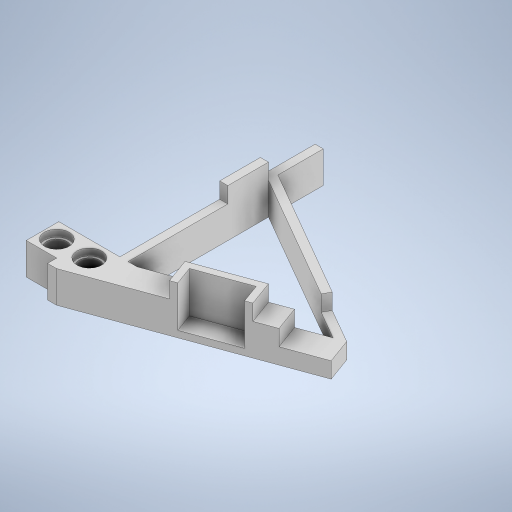
# Autodesk Inventor part: blokerv9
Saved by Autodesk Inventor 2023 (Build 270158000, 158)
## iProperties
Created: 2022-10-20
Part Number: blokerv9
Material: Ogólny
Document SubType Name: Modeling
Designer: kamil
Density: 1 g/cm^3
Appearance: Domyślna
Author: kamil
Autodesk Inventor part; units mm, degrees
ref_plane "YZ Plane" through (0, 0, 0) normal (1, 0, 0) x (0, 1, 0)
ref_plane "XZ Plane" through (0, 0, 0) normal (0, 1, 0) x (-1, 0, 0)
ref_plane "XY Plane" through (0, 0, 0) normal (0, 0, 1) x (1, 0, 0)
sketch "Sketch2" plane through (0, 0, 0) normal (0, 1, 0) x (-1, 0, 0)
  line L0 (7.5, -4) -> (-7.5, -4)
  line L1 (-7.5, -4) -> (-7.5, 4)
  line L2 (-7.5, 4) -> (7.5, 4)
  line L3 (7.5, 4) -> (7.5, -4)
  circle A0 centre (4, 0) radius 2.5
  circle A1 centre (-4, 0) radius 2.5
  line L4 (0, -4) -> (0, 11) construction
  circle A2 centre (0, 11) radius 3.7 construction
  line L5 (-30.3941, -4) -> (1.2655, 7.5231) construction
  line L6 (-17.5, -4) -> (-17.5, 0.6931)
  line L7 (-17.5, 0.6931) -> (0, 7.0625)
  line L8 (0, 7.0625) -> (0, 4)
  line L9 (-17.5, -4) -> (-7.5, -4)
  line L10 (-11.8902, 2.7349) -> (-12.4882, 4.3778) construction
  line L11 (-17.5, 0.6931) -> (-51.6831, -11.7486)
  line L12 (-51.6831, -11.7486) -> (-49.4993, -17.7486)
  circle A3 centre (0, 7.0625) radius 55 construction
  line L13 (0, 14.7) -> (0, 62.0625) construction
  line L14 (-49.4993, -17.7486) -> (-11.7254, -4)
  line L15 (-7.5, -4) -> (-7.5, -41.9969)
  line L16 (-7.5, -41.9969) -> (-49.4993, -17.7486)
  line L17 (-9.5, -4) -> (-9.5, -38.5328)
  line L18 (-9.5, -38.5328) -> (-47.0459, -16.8556)
  line L19 (0, 6.2625) -> (-2.198, 6.2625)
  line L20 (-22.5526, -1.1459) -> (-20.3688, -7.1459)
  line L21 (-20.3688, -7.1459) -> (-35.4039, -12.6183)
  line L22 (-35.4039, -12.6183) -> (-37.5877, -6.6183)
  line L23 (-37.5877, -6.6183) -> (-22.5526, -1.1459)
  line L24 (-9.5, -38.5328) -> (-9.5, -51.9969)
  line L25 (-9.5, -51.9969) -> (-7.5, -51.9969)
  line L26 (-7.5, -51.9969) -> (-7.5, -41.9969)
  arc A4 (0, 47.0625) -> (-37.5877, -6.6183) centre (0, 7.0625) ccw construction
  line L27 (-7.5, -38.5328) -> (-9.5, -38.5328)
  line L28 (-9.5, -38.5328) -> (-9.5, -28.5328)
  line L29 (-9.5, -28.5328) -> (-7.5, -28.5328)
  line L30 (-7.5, -28.5328) -> (-7.5, -38.5328)
  circle A5 centre (4, 0) radius 3.05
  circle A6 centre (-4, 0) radius 3.05
  line L31 (-42.2862, -8.3284) -> (-40.1023, -14.3284)
  line L32 (-40.1023, -20.8645) -> (-41.1023, -22.5965)
  point P0 (0, 0)
  point P1 (7.5, 0)
  point P2 (0, 3.5)
  point P3 (-9.5, -40.8422)
  dimension "d6" = 5
  dimension "d7" = 8
  dimension "d9" = 11
  dimension "d10" = 7.4
  dimension "d11" = 8
  dimension "d12" = 15
  dimension "d13" = 70
  dimension "d14" = 10
  dimension "d21" = 14
  dimension "d25" = 55
  dimension "d27" = 6
  dimension "d35" = 60
  dimension "d36" = 3.5
  dimension "d37" = 2
  dimension "d38" = 2
  dimension "d39" = 0.8
  dimension "d40" = 10
  dimension "d41" = 40
  dimension "d42" = 16
  dimension "d43" = 10
  dimension "d46" = 6.1
  dimension "d47" = 6.1
  dimension "d50" = 10
  constraints: 66 end point, 20 point on line, 12 perpendicular, 8 parallel, 7 centre point, 6 point on circle, 5 coincident, 5 vertical, 4 midpoint, 3 horizontal alignment, 3 vertical alignment, 2 horizontal, 1 collinear, 1 tangent, 1 other
  measures "d6" diameter of A0
  measures "d7" distance of A1.centre A0.centre
  measures "d9" distance of L4.end point (0, 0)
  measures "d10" diameter of A2
  measures "d11" distance of L2.end L0.start
  measures "d12" distance of L0.start L0.end
  measures "d13" angle of L4 L5
  measures "d14" distance of L6.start L0.end
  measures "d21" distance of L10.start L5.end
  measures "d25" distance of L13.end L7.end
  measures "d27" vertical distance of L11.end L12.end
  measures "d35" angle of L16 L15
  measures "d36" horizontal distance of L15.start A1.centre
  measures "d37" distance between parallel lines of L16 L18
  measures "d38" distance between parallel lines of L17 L15
  measures "d39" distance of L7.end L19.start
  measures "d40" distance of L25.end L15.end
  measures "d41" distance of A4.start A4.centre
  measures "d42" distance between parallel lines of L20 L22
  measures "d43" distance of L29.end L27.start
  measures "d46" diameter of A5
  measures "d47" diameter of A6
  measures "d50" distance from line of L11.end L31
extrude "Extrusion1" add sketch "Sketch2" along normal blind 7.8 contours L0 L1 L2 L3 | L9 L6 L7 L19 L8 L2 L1 | L15 L29 L17 L9 | L14 L20 L11 L6 L9 | L15 L16 L24 L27 | L24 L16 L32 L18 | L26 L25 L24 L16 | L14 L31 L11 L22
extrude "Wyciągnięcie proste3" add sketch "Sketch2" along normal blind 11.7 contours L15 L27 L17 L29 | L14 L22 L11 L20
extrude "Wyciągnięcie proste4" add sketch "Sketch2" along normal blind 6.1 contours A5 | A6
extrude "Wyciągnięcie proste5" add sketch "Sketch2" along normal blind 3.9 contours L32 L16 L14 L18 | L14 L12 L11 L31
sketch "Szkic6" plane through (2.198, 0, 6.2625) normal (0.342, 0, 0.9397) x (0.9397, 0, -0.342)
  line L0 (21.661, 11.7) -> (37.661, 11.7) projected
  line L1 (23.261, 11.7) -> (36.061, 11.7)
  line L2 (36.061, 11.7) -> (36.061, 1.6)
  line L3 (36.061, 1.6) -> (23.261, 1.6)
  line L4 (23.261, 1.6) -> (23.261, 11.7)
  line L5 (37.661, 7.8) -> (37.661, 11.7) projected
  line L6 (21.661, 7.8) -> (21.661, 11.7) projected
  line L7 (0, 0) -> (52.661, 0) projected
  point P0 (0.0765, 0)
  point P1 (37.661, 9.75)
  point P2 (21.661, 9.75)
  dimension "d59" = 1.6
  dimension "d60" = 1.6
  dimension "d61" = 1.6
  constraints: 8 end point, 2 midpoint, 2 parallel, 1 horizontal, 1 perpendicular, 1 point on line
  measures "d59" distance from line of point (37.661, 9.75) L2
  measures "d60" distance from line of point (21.661, 9.75) L4
  measures "d61" distance between parallel lines of L7 L3
extrude "Wyciągnięcie proste7" cut sketch "Szkic6" against normal blind 4.785
mirror "Odbij1" [suppressed]
equation "\"d38\" = d37"
equation "\"d47\" = d46"
body "Solid3"
